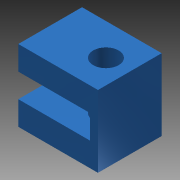
# Autodesk Inventor part: End stop clip
Saved by Autodesk Inventor 2013 SP2 (Build 170200200, 200)
## iProperties
Created: 2017-05-28
Part Number: End stop clip
Material: Generic
Document SubType Name: Modeling
Designer: hdv
Density: 1 g/cm^3
Author: hdv
Autodesk Inventor part; units mm, degrees
ref_plane "YZ Plane" through (0, 0, 0) normal (1, 0, 0) x (0, 1, 0)
ref_plane "XZ Plane" through (0, 0, 0) normal (0, 1, 0) x (-1, 0, 0)
ref_plane "XY Plane" through (0, 0, 0) normal (0, 0, 1) x (1, 0, 0)
sketch "Sketch1" plane through (0, 0, 0) normal (0, 0, 1) x (1, 0, 0)
  line L0 (0, 0) -> (10, 0)
  line L1 (10, 0) -> (10, 3)
  line L2 (10, 3) -> (0, 3)
  line L3 (0, 3) -> (0, 0)
  line L4 (10, 3) -> (9, 3)
  line L5 (9, 3) -> (9, 6)
  line L6 (9, 6) -> (10, 6)
  line L7 (10, 6) -> (10, 3)
  line L8 (10, 6) -> (0, 6)
  line L9 (0, 6) -> (0, 9)
  line L10 (0, 9) -> (10, 9)
  line L11 (10, 9) -> (10, 6)
  dimension "d0" = 3
  dimension "d1" = 10
  dimension "d2" = 3
  dimension "d3" = 3
  dimension "d4" = 1
  constraints: 24 end point, 6 parallel, 3 horizontal, 3 perpendicular, 1 collinear
  measures "d0" distance of L2.end L0.start
  measures "d1" distance of L0.start L0.end
  measures "d2" distance of L6.end L1.end
  measures "d3" distance of L9.end L8.end
  measures "d4" distance between parallel lines of L7 L5
extrude "Extrusion1" add sketch "Sketch1" along normal blind 8
sketch "Sketch2" plane through (0, 0, 0) normal (0, -1, 0) x (1, 0, 0)
  line L0 (10, 0) -> (10, 8) projected
  circle A0 centre (7, 4) radius 1.6
  point P0 (10, 4)
  dimension "d7" = 3.2
  dimension "d8" = 3
  constraints: 1 centre point, 1 horizontal alignment, 1 midpoint
  measures "d7" diameter of A0
  measures "d8" distance from line of L0 A0.centre
extrude "Extrusion2" cut sketch "Sketch2" against normal blind 10
body "Solid1"
